Autodesk Fusion 360 part; units mm, degrees
(part 8 of 8)
sketch "Sketch1 (2)" plane through (0, 0, 0) normal (0, 0, 1) x (1, 0, 0) in component "Component"
  spline S0 degree 5 poles (13.0648, -1.7938) (13.065, -1.7938) (13.0653, -1.7938) (13.0658, -1.7939) (13.0667, -1.794) (13.0679, -1.7941) (13.0693, -1.7943) (13.071, -1.7944) (13.0728, -1.7946) (13.0748, -1.7948) (13.077, -1.795) (13.0793, -1.7952) (13.0819, -1.7955) (13.0846, -1.7957) (13.0874, -1.7959) (13.0905, -1.7961) (13.0937, -1.7964) (13.0971, -1.7966) (13.1006, -1.7968) (13.1043, -1.797) (13.1081, -1.7972) (13.1121, -1.7975) (13.1162, -1.7977) (13.1205, -1.7978) (13.1249, -1.798) (13.1295, -1.7982) (13.1342, -1.7984) (13.1391, -1.7985) (13.1441, -1.7987) (13.1492, -1.7988) (13.1544, -1.7989) (13.1598, -1.799) (13.1653, -1.7991) (13.171, -1.7991) (13.1767, -1.7992) (13.1826, -1.7992) (13.1886, -1.7992) (13.1948, -1.7992) (13.201, -1.7991) (13.2074, -1.7991) (13.2139, -1.799) (13.2205, -1.7989) (13.2272, -1.7987) (13.2341, -1.7986) (13.241, -1.7984) (13.2481, -1.7982) (13.2552, -1.798) (13.2625, -1.7977) (13.2699, -1.7974) (13.2774, -1.7971) (13.285, -1.7968) (13.2927, -1.7964) (13.3004, -1.796) (13.3083, -1.7955) (13.3163, -1.7951) (13.3244, -1.7946) (13.3326, -1.7941) (13.3409, -1.7935) (13.3493, -1.7929) (13.3578, -1.7923) (13.3663, -1.7916) (13.375, -1.7909) (13.3838, -1.7902) (13.3926, -1.7895) (13.4015, -1.7887) (13.4106, -1.7878) (13.4197, -1.787) (13.4289, -1.7861) (13.4382, -1.7851) (13.4475, -1.7842) (13.457, -1.7832) (13.4665, -1.7821) (13.4762, -1.781) (13.4859, -1.7799) (13.4957, -1.7787) (13.5055, -1.7775) (13.5155, -1.7763) (13.5255, -1.775) (13.5356, -1.7737) (13.5458, -1.7723) (13.5561, -1.7709) (13.5664, -1.7695) (13.5768, -1.768) (13.5873, -1.7665) (13.5978, -1.7649) (13.6085, -1.7633) (13.6192, -1.7616) (13.63, -1.7599) (13.6408, -1.7582) (13.6517, -1.7564) (13.6627, -1.7546) (13.6738, -1.7527) (13.6849, -1.7508) (13.6961, -1.7489) (13.7074, -1.7469) (13.7187, -1.7448) (13.7301, -1.7428) (13.7415, -1.7406) (13.7531, -1.7384) (13.7647, -1.7362) (13.7763, -1.734) (13.788, -1.7316) (13.7998, -1.7293) (13.8117, -1.7269) (13.8236, -1.7244) (13.8355, -1.7219) (13.8476, -1.7194) (13.8596, -1.7168) (13.8718, -1.7142) (13.884, -1.7115) (13.8963, -1.7088) (13.9086, -1.706) (13.921, -1.7032) (13.9334, -1.7003) (13.9459, -1.6974) (13.9584, -1.6944) (13.971, -1.6914) (13.9837, -1.6883) (13.9964, -1.6852) (14.0092, -1.682) (14.022, -1.6788) (14.0349, -1.6755) (14.0478, -1.6722) (14.0608, -1.6689) (14.0738, -1.6655) (14.0869, -1.662) (14.1, -1.6585) (14.1132, -1.6549) (14.1264, -1.6513) (14.1397, -1.6476) (14.153, -1.6439) (14.1664, -1.6402) (14.1798, -1.6364) (14.1933, -1.6325) (14.2068, -1.6286) (14.2204, -1.6246) (14.234, -1.6206) (14.2476, -1.6165) (14.2613, -1.6124) (14.2751, -1.6082) (14.2889, -1.604) (14.3027, -1.5998) (14.3166, -1.5954) (14.3305, -1.5911) (14.3445, -1.5866) (14.3585, -1.5821) (14.3725, -1.5776) (14.3866, -1.573) (14.4007, -1.5684) (14.4149, -1.5637) (14.4291, -1.559) (14.4434, -1.5542) (14.4577, -1.5493) (14.472, -1.5444) (14.4864, -1.5395) (14.5008, -1.5344) (14.5152, -1.5294) (14.5297, -1.5243) (14.5442, -1.5191) (14.5588, -1.5139) (14.5734, -1.5086) (14.588, -1.5033) (14.6027, -1.4979) (14.6174, -1.4925) (14.6322, -1.487) (14.6469, -1.4814) (14.6617, -1.4758) (14.6766, -1.4702) (14.6915, -1.4645) (14.7064, -1.4587) (14.7213, -1.4529) (14.7363, -1.4471) (14.7513, -1.4411) (14.7664, -1.4352) (14.7814, -1.4291) (14.7965, -1.4231) (14.8117, -1.4169) (14.8269, -1.4107) (14.8421, -1.4045) (14.8573, -1.3982) (14.8725, -1.3918) (14.8878, -1.3854) (14.9032, -1.3789) (14.9185, -1.3724) (14.9339, -1.3659) (14.9493, -1.3592) (14.9647, -1.3525) (14.9802, -1.3458) (14.9957, -1.339) (15.0112, -1.3322) (15.0267, -1.3252) (15.0423, -1.3183) (15.0579, -1.3113) (15.0735, -1.3042) (15.0892, -1.2971) (15.1049, -1.2899) (15.1206, -1.2827) (15.1363, -1.2754) (15.152, -1.268) (15.1678, -1.2606) (15.1836, -1.2532) (15.1994, -1.2456) (15.2153, -1.2381) (15.2311, -1.2304) (15.247, -1.2228) (15.2629, -1.215) (15.2789, -1.2072) (15.2948, -1.1994) (15.3108, -1.1915) (15.3268, -1.1835) (15.3428, -1.1755) (15.3589, -1.1674) (15.3749, -1.1593) (15.391, -1.1511) (15.4071, -1.1429) (15.4232, -1.1346) (15.4394, -1.1262) (15.4555, -1.1178) (15.4717, -1.1094) (15.4879, -1.1008) (15.5041, -1.0923) (15.5204, -1.0836) (15.5366, -1.0749) (15.5529, -1.0662) (15.5692, -1.0574) (15.5855, -1.0485) (15.6018, -1.0396) (15.6182, -1.0307) (15.6345, -1.0216) (15.6509, -1.0126) (15.6673, -1.0034) (15.6837, -0.9942) (15.7001, -0.985) (15.7165, -0.9757) (15.733, -0.9663) (15.7495, -0.9569) (15.7659, -0.9474) (15.7824, -0.9379) (15.7989, -0.9283) (15.8154, -0.9187) (15.832, -0.909) (15.8452, -0.9012) (15.8552, -0.8953) (15.8618, -0.8913) (15.8651, -0.8894) knots 0 0 0 0 0 0 0.00416667 0.00833333 0.0125 0.01666667 0.02083333 0.025 0.02916667 0.03333333 0.0375 0.04166667 0.04583333 0.05 0.05416667 0.05833333 0.0625 0.06666667 0.07083333 0.075 0.07916667 0.08333333 0.0875 0.09166667 0.09583333 0.1 0.10416667 0.10833333 0.1125 0.11666667 0.12083333 0.125 0.12916667 0.13333333 0.1375 0.14166667 0.14583333 0.15 0.15416667 0.15833333 0.1625 0.16666667 0.17083333 0.175 0.17916667 0.18333333 0.1875 0.19166667 0.19583333 0.2 0.20416667 0.20833333 0.2125 0.21666667 0.22083333 0.225 0.22916667 0.23333333 0.2375 0.24166667 0.24583333 0.25 0.25416667 0.25833333 0.2625 0.26666667 0.27083333 0.275 0.27916667 0.28333333 0.2875 0.29166667 0.29583333 0.3 0.30416667 0.30833333 0.3125 0.31666667 0.32083333 0.325 0.32916667 0.33333333 0.3375 0.34166667 0.34583333 0.35 0.35416667 0.35833333 0.3625 0.36666667 0.37083333 0.375 0.37916667 0.38333333 0.3875 0.39166667 0.39583333 0.4 0.40416667 0.40833333 0.4125 0.41666667 0.42083333 0.425 0.42916667 0.43333333 0.4375 0.44166667 0.44583333 0.45 0.45416667 0.45833333 0.4625 0.46666667 0.47083333 0.475 0.47916667 0.48333333 0.4875 0.49166667 0.49583333 0.5 0.50416667 0.50833333 0.5125 0.51666667 0.52083333 0.525 0.52916667 0.53333333 0.5375 0.54166667 0.54583333 0.55 0.55416667 0.55833333 0.5625 0.56666667 0.57083333 0.575 0.57916667 0.58333333 0.5875 0.59166667 0.59583333 0.6 0.60416667 0.60833333 0.6125 0.61666667 0.62083333 0.625 0.62916667 0.63333333 0.6375 0.64166667 0.64583333 0.65 0.65416667 0.65833333 0.6625 0.66666667 0.67083333 0.675 0.67916667 0.68333333 0.6875 0.69166667 0.69583333 0.7 0.70416667 0.70833333 0.7125 0.71666667 0.72083333 0.725 0.72916667 0.73333333 0.7375 0.74166667 0.74583333 0.75 0.75416667 0.75833333 0.7625 0.76666667 0.77083333 0.775 0.77916667 0.78333333 0.7875 0.79166667 0.79583333 0.8 0.80416667 0.80833333 0.8125 0.81666667 0.82083333 0.825 0.82916667 0.83333333 0.8375 0.84166667 0.84583333 0.85 0.85416667 0.85833333 0.8625 0.86666667 0.87083333 0.875 0.87916667 0.88333333 0.8875 0.89166667 0.89583333 0.9 0.90416667 0.90833333 0.9125 0.91666667 0.92083333 0.925 0.92916667 0.93333333 0.9375 0.94166667 0.94583333 0.95 0.95416667 0.95833333 0.9625 0.96666667 0.97083333 0.975 0.97916667 0.98333333 0.9875 0.99166667 0.99583333 1 1 1 1 1 1
  spline S1 degree 5 poles (13.0648, 1.7938) (13.065, 1.7938) (13.0653, 1.7938) (13.0658, 1.7939) (13.0667, 1.794) (13.0679, 1.7941) (13.0693, 1.7943) (13.071, 1.7944) (13.0728, 1.7946) (13.0748, 1.7948) (13.077, 1.795) (13.0793, 1.7952) (13.0819, 1.7955) (13.0846, 1.7957) (13.0874, 1.7959) (13.0905, 1.7961) (13.0937, 1.7964) (13.0971, 1.7966) (13.1006, 1.7968) (13.1043, 1.797) (13.1081, 1.7972) (13.1121, 1.7975) (13.1162, 1.7977) (13.1205, 1.7978) (13.1249, 1.798) (13.1295, 1.7982) (13.1342, 1.7984) (13.1391, 1.7985) (13.1441, 1.7987) (13.1492, 1.7988) (13.1544, 1.7989) (13.1598, 1.799) (13.1653, 1.7991) (13.171, 1.7991) (13.1767, 1.7992) (13.1826, 1.7992) (13.1886, 1.7992) (13.1948, 1.7992) (13.201, 1.7991) (13.2074, 1.7991) (13.2139, 1.799) (13.2205, 1.7989) (13.2272, 1.7987) (13.2341, 1.7986) (13.241, 1.7984) (13.2481, 1.7982) (13.2552, 1.798) (13.2625, 1.7977) (13.2699, 1.7974) (13.2774, 1.7971) (13.285, 1.7968) (13.2927, 1.7964) (13.3004, 1.796) (13.3083, 1.7955) (13.3163, 1.7951) (13.3244, 1.7946) (13.3326, 1.7941) (13.3409, 1.7935) (13.3493, 1.7929) (13.3578, 1.7923) (13.3663, 1.7916) (13.375, 1.7909) (13.3838, 1.7902) (13.3926, 1.7895) (13.4015, 1.7887) (13.4106, 1.7878) (13.4197, 1.787) (13.4289, 1.7861) (13.4382, 1.7851) (13.4475, 1.7842) (13.457, 1.7832) (13.4665, 1.7821) (13.4762, 1.781) (13.4859, 1.7799) (13.4957, 1.7787) (13.5055, 1.7775) (13.5155, 1.7763) (13.5255, 1.775) (13.5356, 1.7737) (13.5458, 1.7723) (13.5561, 1.7709) (13.5664, 1.7695) (13.5768, 1.768) (13.5873, 1.7665) (13.5978, 1.7649) (13.6085, 1.7633) (13.6192, 1.7616) (13.63, 1.7599) (13.6408, 1.7582) (13.6517, 1.7564) (13.6627, 1.7546) (13.6738, 1.7527) (13.6849, 1.7508) (13.6961, 1.7489) (13.7074, 1.7469) (13.7187, 1.7448) (13.7301, 1.7428) (13.7415, 1.7406) (13.7531, 1.7384) (13.7647, 1.7362) (13.7763, 1.734) (13.788, 1.7316) (13.7998, 1.7293) (13.8117, 1.7269) (13.8236, 1.7244) (13.8355, 1.7219) (13.8476, 1.7194) (13.8596, 1.7168) (13.8718, 1.7142) (13.884, 1.7115) (13.8963, 1.7088) (13.9086, 1.706) (13.921, 1.7032) (13.9334, 1.7003) (13.9459, 1.6974) (13.9584, 1.6944) (13.971, 1.6914) (13.9837, 1.6883) (13.9964, 1.6852) (14.0092, 1.682) (14.022, 1.6788) (14.0349, 1.6755) (14.0478, 1.6722) (14.0608, 1.6689) (14.0738, 1.6655) (14.0869, 1.662) (14.1, 1.6585) (14.1132, 1.6549) (14.1264, 1.6513) (14.1397, 1.6476) (14.153, 1.6439) (14.1664, 1.6402) (14.1798, 1.6364) (14.1933, 1.6325) (14.2068, 1.6286) (14.2204, 1.6246) (14.234, 1.6206) (14.2476, 1.6165) (14.2613, 1.6124) (14.2751, 1.6082) (14.2889, 1.604) (14.3027, 1.5998) (14.3166, 1.5954) (14.3305, 1.5911) (14.3445, 1.5866) (14.3585, 1.5821) (14.3725, 1.5776) (14.3866, 1.573) (14.4007, 1.5684) (14.4149, 1.5637) (14.4291, 1.559) (14.4434, 1.5542) (14.4577, 1.5493) (14.472, 1.5444) (14.4864, 1.5395) (14.5008, 1.5344) (14.5152, 1.5294) (14.5297, 1.5243) (14.5442, 1.5191) (14.5588, 1.5139) (14.5734, 1.5086) (14.588, 1.5033) (14.6027, 1.4979) (14.6174, 1.4925) (14.6322, 1.487) (14.6469, 1.4814) (14.6617, 1.4758) (14.6766, 1.4702) (14.6915, 1.4645) (14.7064, 1.4587) (14.7213, 1.4529) (14.7363, 1.4471) (14.7513, 1.4411) (14.7664, 1.4352) (14.7814, 1.4291) (14.7965, 1.4231) (14.8117, 1.4169) (14.8269, 1.4107) (14.8421, 1.4045) (14.8573, 1.3982) (14.8725, 1.3918) (14.8878, 1.3854) (14.9032, 1.3789) (14.9185, 1.3724) (14.9339, 1.3659) (14.9493, 1.3592) (14.9647, 1.3525) (14.9802, 1.3458) (14.9957, 1.339) (15.0112, 1.3322) (15.0267, 1.3252) (15.0423, 1.3183) (15.0579, 1.3113) (15.0735, 1.3042) (15.0892, 1.2971) (15.1049, 1.2899) (15.1206, 1.2827) (15.1363, 1.2754) (15.152, 1.268) (15.1678, 1.2606) (15.1836, 1.2532) (15.1994, 1.2456) (15.2153, 1.2381) (15.2311, 1.2304) (15.247, 1.2228) (15.2629, 1.215) (15.2789, 1.2072) (15.2948, 1.1994) (15.3108, 1.1915) (15.3268, 1.1835) (15.3428, 1.1755) (15.3589, 1.1674) (15.3749, 1.1593) (15.391, 1.1511) (15.4071, 1.1429) (15.4232, 1.1346) (15.4394, 1.1262) (15.4555, 1.1178) (15.4717, 1.1094) (15.4879, 1.1008) (15.5041, 1.0923) (15.5204, 1.0836) (15.5366, 1.0749) (15.5529, 1.0662) (15.5692, 1.0574) (15.5855, 1.0485) (15.6018, 1.0396) (15.6182, 1.0307) (15.6345, 1.0216) (15.6509, 1.0126) (15.6673, 1.0034) (15.6837, 0.9942) (15.7001, 0.985) (15.7165, 0.9757) (15.733, 0.9663) (15.7495, 0.9569) (15.7659, 0.9474) (15.7824, 0.9379) (15.7989, 0.9283) (15.8154, 0.9187) (15.832, 0.909) (15.8452, 0.9012) (15.8552, 0.8953) (15.8618, 0.8913) (15.8651, 0.8894) knots 0 0 0 0 0 0 0.00416667 0.00833333 0.0125 0.01666667 0.02083333 0.025 0.02916667 0.03333333 0.0375 0.04166667 0.04583333 0.05 0.05416667 0.05833333 0.0625 0.06666667 0.07083333 0.075 0.07916667 0.08333333 0.0875 0.09166667 0.09583333 0.1 0.10416667 0.10833333 0.1125 0.11666667 0.12083333 0.125 0.12916667 0.13333333 0.1375 0.14166667 0.14583333 0.15 0.15416667 0.15833333 0.1625 0.16666667 0.17083333 0.175 0.17916667 0.18333333 0.1875 0.19166667 0.19583333 0.2 0.20416667 0.20833333 0.2125 0.21666667 0.22083333 0.225 0.22916667 0.23333333 0.2375 0.24166667 0.24583333 0.25 0.25416667 0.25833333 0.2625 0.26666667 0.27083333 0.275 0.27916667 0.28333333 0.2875 0.29166667 0.29583333 0.3 0.30416667 0.30833333 0.3125 0.31666667 0.32083333 0.325 0.32916667 0.33333333 0.3375 0.34166667 0.34583333 0.35 0.35416667 0.35833333 0.3625 0.36666667 0.37083333 0.375 0.37916667 0.38333333 0.3875 0.39166667 0.39583333 0.4 0.40416667 0.40833333 0.4125 0.41666667 0.42083333 0.425 0.42916667 0.43333333 0.4375 0.44166667 0.44583333 0.45 0.45416667 0.45833333 0.4625 0.46666667 0.47083333 0.475 0.47916667 0.48333333 0.4875 0.49166667 0.49583333 0.5 0.50416667 0.50833333 0.5125 0.51666667 0.52083333 0.525 0.52916667 0.53333333 0.5375 0.54166667 0.54583333 0.55 0.55416667 0.55833333 0.5625 0.56666667 0.57083333 0.575 0.57916667 0.58333333 0.5875 0.59166667 0.59583333 0.6 0.60416667 0.60833333 0.6125 0.61666667 0.62083333 0.625 0.62916667 0.63333333 0.6375 0.64166667 0.64583333 0.65 0.65416667 0.65833333 0.6625 0.66666667 0.67083333 0.675 0.67916667 0.68333333 0.6875 0.69166667 0.69583333 0.7 0.70416667 0.70833333 0.7125 0.71666667 0.72083333 0.725 0.72916667 0.73333333 0.7375 0.74166667 0.74583333 0.75 0.75416667 0.75833333 0.7625 0.76666667 0.77083333 0.775 0.77916667 0.78333333 0.7875 0.79166667 0.79583333 0.8 0.80416667 0.80833333 0.8125 0.81666667 0.82083333 0.825 0.82916667 0.83333333 0.8375 0.84166667 0.84583333 0.85 0.85416667 0.85833333 0.8625 0.86666667 0.87083333 0.875 0.87916667 0.88333333 0.8875 0.89166667 0.89583333 0.9 0.90416667 0.90833333 0.9125 0.91666667 0.92083333 0.925 0.92916667 0.93333333 0.9375 0.94166667 0.94583333 0.95 0.95416667 0.95833333 0.9625 0.96666667 0.97083333 0.975 0.97916667 0.98333333 0.9875 0.99166667 0.99583333 1 1 1 1 1 1
  spline S2 degree 5 poles (13.0636, -1.7936) (13.0637, -1.7936) (13.0638, -1.7936) (13.0639, -1.7936) (13.0641, -1.7937) (13.0644, -1.7937) (13.0646, -1.7937) (13.0647, -1.7937) (13.0648, -1.7938) (13.0648, -1.7938) knots 0 0 0 0 0 0 0.2 0.4 0.6 0.8 1 1 1 1 1 1
  spline S3 degree 5 poles (13.0636, 1.7936) (13.0637, 1.7936) (13.0638, 1.7936) (13.0639, 1.7936) (13.0641, 1.7937) (13.0644, 1.7937) (13.0646, 1.7937) (13.0647, 1.7937) (13.0648, 1.7938) (13.0648, 1.7938) knots 0 0 0 0 0 0 0.2 0.4 0.6 0.8 1 1 1 1 1 1
  line L0 (0, 0) -> (13.0636, -1.7936)
  line L1 (0, 0) -> (13.0636, 1.7936)
  arc A0 (15.8651, -0.8894) -> (15.8651, 0.8894) centre (0, 0) ccw
  point P0 (13.0685, -1.7942)
  point P1 (13.0747, -1.7948)
  point P2 (13.0834, -1.7956)
  point P3 (13.0945, -1.7964)
  point P4 (13.1082, -1.7972)
  point P5 (13.1243, -1.798)
  point P6 (13.1429, -1.7986)
  point P7 (13.164, -1.799)
  point P8 (13.1876, -1.7992)
  point P9 (13.2137, -1.799)
  point P10 (13.2422, -1.7984)
  point P11 (13.2732, -1.7973)
  point P12 (13.3067, -1.7956)
  point P13 (13.3426, -1.7934)
  point P14 (13.381, -1.7904)
  point P15 (13.4218, -1.7868)
  point P16 (13.465, -1.7823)
  point P17 (13.5107, -1.7769)
  point P18 (13.5587, -1.7705)
  point P19 (13.609, -1.7632)
  point P20 (13.6618, -1.7548)
  point P21 (13.7168, -1.7452)
  point P22 (13.7742, -1.7344)
  point P23 (13.8338, -1.7223)
  point P24 (13.8957, -1.7089)
  point P25 (13.9598, -1.6941)
  point P26 (14.0261, -1.6778)
  point P27 (14.0946, -1.6599)
  point P28 (14.1652, -1.6405)
  point P29 (14.2379, -1.6194)
  point P30 (14.3128, -1.5966)
  point P31 (14.3896, -1.572)
  point P32 (14.4685, -1.5456)
  point P33 (14.5494, -1.5173)
  point P34 (14.6321, -1.487)
  point P35 (14.7168, -1.4547)
  point P36 (14.8034, -1.4203)
  point P37 (14.8917, -1.3838)
  point P38 (14.9818, -1.3451)
  point P39 (15.0737, -1.3041)
  point P40 (15.1672, -1.2609)
  point P41 (15.2624, -1.2153)
  point P42 (15.3592, -1.1673)
  point P43 (15.4575, -1.1168)
  point P44 (15.5573, -1.0638)
  point P45 (15.6585, -1.0083)
  point P46 (15.7611, -0.9502)
  point P47 (13.0685, 1.7942)
  point P48 (13.0747, 1.7948)
  point P49 (13.0834, 1.7956)
  point P50 (13.0945, 1.7964)
  point P51 (13.1082, 1.7972)
  point P52 (13.1243, 1.798)
  point P53 (13.1429, 1.7986)
  point P54 (13.164, 1.799)
  point P55 (13.1876, 1.7992)
  point P56 (13.2137, 1.799)
  point P57 (13.2422, 1.7984)
  point P58 (13.2732, 1.7973)
  point P59 (13.3067, 1.7956)
  point P60 (13.3426, 1.7934)
  point P61 (13.381, 1.7904)
  point P62 (13.4218, 1.7868)
  point P63 (13.465, 1.7823)
  point P64 (13.5107, 1.7769)
  point P65 (13.5587, 1.7705)
  point P66 (13.609, 1.7632)
  point P67 (13.6618, 1.7548)
  point P68 (13.7168, 1.7452)
  point P69 (13.7742, 1.7344)
  point P70 (13.8338, 1.7223)
  point P71 (13.8957, 1.7089)
  point P72 (13.9598, 1.6941)
  point P73 (14.0261, 1.6778)
  point P74 (14.0946, 1.6599)
  point P75 (14.1652, 1.6405)
  point P76 (14.2379, 1.6194)
  point P77 (14.3128, 1.5966)
  point P78 (14.3896, 1.572)
  point P79 (14.4685, 1.5456)
  point P80 (14.5494, 1.5173)
  point P81 (14.6321, 1.487)
  point P82 (14.7168, 1.4547)
  point P83 (14.8034, 1.4203)
  point P84 (14.8917, 1.3838)
  point P85 (14.9818, 1.3451)
  point P86 (15.0737, 1.3041)
  point P87 (15.1672, 1.2609)
  point P88 (15.2624, 1.2153)
  point P89 (15.3592, 1.1673)
  point P90 (15.4575, 1.1168)
  point P91 (15.5573, 1.0638)
  point P92 (15.6585, 1.0083)
  point P93 (15.7611, 0.9502)
sketch "Sketch2" plane through (0, 0, 0) normal (0, 0, 1) x (1, 0, 0) in component "Component"
  circle A0 centre (0, 0) radius 10.7825
extrude "Extrude1" add sketch "Sketch2" along normal blind 6 makes body 1 in component "Component"
extrude "Extrude2" add sketch "Sketch1 (2)" along normal blind 6 separate body makes body 2 in component "Component"
pattern_circular "C-Pattern1" count 12 over 360 about axis through (0, 0, 1.75) along (0, 0, 1) of "Extrude2" makes body 3 at (4.0705, 1.6597, 2) makes body 4 at (2.6953, 3.4725, 2) makes body 5 at (0.5979, 4.3549, 2) makes body 6 at (-1.6597, 4.0705, 2) makes body 7 at (-4.0705, 1.6597, 2) makes body 8 at (-4.3549, 0.5979, 2) makes body 9 at (-4.0705, -1.6597, 2) makes body 10 at (-2.6953, -3.4725, 2) makes body 11 at (-0.5979, -4.3549, 2) makes body 12 at (2.6953, -3.4725, 2) makes body 13 at (3.4725, -2.6953, 2) in component "Component"
combine "Combine1" operation add target body 1 tool bodies 2 3 4 5 6 7 8 9 10 11 12 13 in component "Component"
sketch "Sketch3" plane through (0, 0, 0) normal (0, 0, 1) x (1, 0, 0) in component "Component"
  line L0 (0, 0) -> (49.8984, 0) construction
  line L1 (49.8984, 0) -> (49.8984, 3) construction
  line L2 (49.8984, 3) -> (0, 3) construction
  line L3 (0, 3) -> (0, 0) construction
  constraint perpendicular L0 L1
  constraint parallel L0 L2
  constraint parallel L1 L3
extrude "Extrude3" cut sketch "Sketch1" against normal blind 6 contours A24 | A25 | A26 | A27 bodies 1 in component "Component"
component "Component" placed x (1, 0, 0) y (0, 1, 0) z (0, 0, 1) at (0, 0, 0)
component "Component" placed x (1, 0, 0) y (0, 1, 0) z (0, 0, 1) at (34, 0, 0)

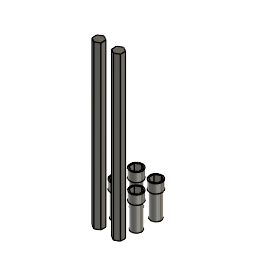
design "card-shuffler-hex-shaft-and-connectors"
part number: 2026-07-29-21-30-18-226
part number: 2026-07-29-22-06-59-016
part number: 2026-07-29-22-06-59-022
part number: 2026-07-29-22-06-59-026
Autodesk Fusion 360 part; units mm, degrees
sketch "Sketch1" plane through (0, 0, 0) normal (0, 0, 1) x (1, 0, 0)
  line L0 (-2.5, -1.4434) -> (0, -2.8868)
  line L1 (0, -2.8868) -> (2.5, -1.4434)
  line L2 (2.5, -1.4434) -> (2.5, 1.4434)
  line L3 (2.5, 1.4434) -> (0, 2.8868)
  line L4 (0, 2.8868) -> (-2.5, 1.4434)
  line L5 (-2.5, 1.4434) -> (-2.5, -1.4434)
  line L6 (-2.65, 8.47) -> (0, 6.94)
  line L7 (0, 6.94) -> (2.65, 8.47)
  line L8 (2.65, 8.47) -> (2.65, 11.53)
  line L9 (2.65, 11.53) -> (0, 13.06)
  line L10 (0, 13.06) -> (-2.65, 11.53)
  line L11 (-2.65, 11.53) -> (-2.65, 8.47)
  circle A0 centre (0, 10) radius 3.5
  point P0 (0, 10)
  dimension "d3" = 2.5
  dimension "d4" = 2.65
  dimension "d5" = 7
  constraint coincident P0 A0.centre
  measures "d3" distance of origin L5
  measures "d4" distance of P0 L11
  measures "d5" diameter of A0
extrude "Extrude1" add sketch "Sketch1" along normal blind 5 contours A0 makes body 1
extrude "Extrude2" add sketch "Sketch1" along normal blind 1 contours L6 L7 L8 L9 L10 L11 bodies 1
sketch "Sketch2" plane through (0, 0, 0) normal (0, 0, 1) x (1, 0, 0)
  circle A0 centre (0, 10) radius 2.9
  dimension "d10" = 5.8
  measures "d10" diameter of A0
extrude "Extrude3" add sketch "Sketch2" against normal blind 14 bodies 1
extrude "Extrude4" add sketch "Sketch1" along normal blind 91 separate body contours L0 L1 L2 L3 L4 L5 makes body 2
move_body "Move1" bodies 1 to x (1, 0, 0) y (0, 1, 0) z (0, 0, 1) at (0, 0, 13)
copy_body "CopyPasteBodies1" bodies 1 makes body 3
move_body "Move2" bodies 3 to x (1, 0, 0) y (0, 1, 0) z (0, 0, 1) at (0, 11, 0)
copy_body "Body->Comp1" bodies 3 removing the originals makes body 4 in component "Component"
copy_body "Body->Comp2" bodies 1 removing the originals makes body 5 in component "Component'"
copy_body "Body->Comp3" bodies 2 removing the originals makes body 6 in component "Component''"
component "Component" placed x (1, 0, 0) y (0, 1, 0) z (0, 0, 1) at (0, 0, 0)
component "Component'" placed x (1, 0, 0) y (0, 1, 0) z (0, 0, 1) at (0, 0, 0)
component "Component''" placed x (1, 0, 0) y (0, 1, 0) z (0, 0, 1) at (0, 0, 0)
component "Component" placed x (1, 0, 0) y (0, 1, 0) z (0, 0, 1) at (-11, 0, 0)
component "Component'" placed x (1, 0, 0) y (0, 1, 0) z (0, 0, 1) at (-11, 0, 0)
component "Component''" placed x (1, 0, 0) y (0, 1, 0) z (0, 0, 1) at (-11, 0, 0)

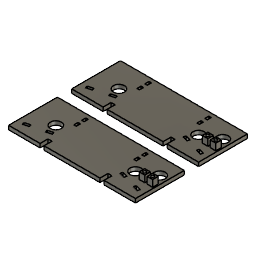
design "card-shuffler-side-plates"
part number: 2026-07-14-13-37-18-342
part number: 2026-07-29-15-30-40-937
Autodesk Fusion 360 part; units mm, degrees
sketch "Sketch1" plane through (0, 0, 0) normal (0, 0, 1) x (1, 0, 0)
  line L0 (0, 0) -> (81, 0)
  line L1 (81, 0) -> (81, 103)
  line L2 (81, 103) -> (0, 103)
  line L3 (0, 103) -> (0, 0)
  line L4 (76, 98) -> (5, 98)
  line L5 (5, 98) -> (5, 5)
  line L6 (5, 5) -> (76, 5)
  line L7 (76, 5) -> (76, 98)
  line L8 (76, 98) -> (5, 5) construction
  line L9 (5, 98) -> (76, 5) construction
  line L10 (81, 0) -> (121, 0)
  line L11 (121, 0) -> (121, 5)
  line L12 (121, 5) -> (81, 5)
  line L13 (81, 5) -> (81, 0)
  line L14 (0, 0) -> (-40, 0)
  line L15 (-40, 0) -> (-40, 5)
  line L16 (-40, 5) -> (0, 5)
  line L17 (0, 5) -> (0, 0)
  line L18 (81, 103) -> (121, 103)
  line L19 (121, 103) -> (121, 98)
  line L20 (121, 98) -> (81, 98)
  line L21 (81, 98) -> (81, 103)
  line L22 (0, 103) -> (-40, 103)
  line L23 (-40, 103) -> (-40, 98)
  line L24 (-40, 98) -> (0, 98)
  line L25 (0, 98) -> (0, 103)
  line L26 (76, 51.5) -> (76, 45)
  line L27 (76, 45) -> (81, 45)
  line L28 (81, 45) -> (81, 58)
  line L29 (81, 58) -> (76, 58)
  line L30 (76, 58) -> (76, 45)
  line L31 (0, 58) -> (5, 58)
  line L32 (5, 58) -> (5, 45)
  line L33 (5, 45) -> (0, 45)
  line L34 (0, 45) -> (0, 58)
  line L35 (81, 98) -> (121, 98)
  line L36 (121, 98) -> (121, 5)
  line L37 (121, 5) -> (81, 5)
  line L38 (81, 5) -> (81, 98)
  line L39 (-40, 98) -> (0, 98)
  line L40 (0, 98) -> (0, 5)
  line L41 (0, 5) -> (-40, 5)
  line L42 (-40, 5) -> (-40, 98)
  line L43 (76, 58) -> (108, 58)
  line L44 (108, 58) -> (108, 45)
  line L45 (108, 45) -> (76, 45)
  line L46 (76, 45) -> (76, 58)
  line L47 (5, 45) -> (-27, 45)
  line L48 (-27, 45) -> (-27, 58)
  line L49 (-27, 58) -> (5, 58)
  line L50 (5, 58) -> (5, 45)
  line L51 (76, 98) -> (81, 98)
  line L52 (5, 98) -> (0, 98)
  line L53 (0, 5) -> (5, 5)
  line L54 (76, 5) -> (81, 5)
  point P0 (40.5, 51.5)
  dimension "d1" = 81
  dimension "d2" = 103
  dimension "d3" = 71
  dimension "d4" = 93
  dimension "d7" = 6.5
  dimension "d8" = 32
  dimension "d9" = 13
  dimension "d14" = 40
  dimension "d15" = 40
  dimension "d16" = 40
  dimension "d17" = 40
  constraint horizontal L0
  constraint vertical L1
  constraint horizontal L2
  constraint vertical L3
  constraint coincident L0.start L3.end
  constraint horizontal L4
  constraint perpendicular L4 L5
  constraint parallel L4 L6
  constraint parallel L5 L7
  constraint coincident L8 P0
  constraint coincident L9 P0
  constraint horizontal L10
  constraint vertical L11
  constraint horizontal L12
  constraint vertical L13
  constraint horizontal L14
  constraint vertical L15
  constraint horizontal L16
  constraint vertical L17
  constraint horizontal L18
  constraint vertical L19
  constraint horizontal L20
  constraint vertical L21
  constraint horizontal L22
  constraint vertical L23
  constraint horizontal L24
  constraint vertical L25
  constraint midpoint L7 L26.start
  constraint parallel L7 L26
  constraint horizontal L27
  constraint vertical L28
  constraint horizontal L29
  constraint vertical L30
  constraint coincident L1 L28.end
  constraint horizontal L31
  constraint vertical L32
  constraint horizontal L33
  constraint vertical L34
  constraint coincident L5 L32.end
  constraint coincident L3 L31.start
  constraint horizontal L35
  constraint vertical L36
  constraint horizontal L37
  constraint vertical L38
  constraint horizontal L39
  constraint vertical L40
  constraint horizontal L41
  constraint vertical L42
  constraint horizontal L43
  constraint vertical L44
  constraint horizontal L45
  constraint vertical L46
  constraint horizontal L47
  constraint vertical L48
  constraint horizontal L49
  constraint vertical L50
  measures "d1" distance of L0.start L0.end
  measures "d2" distance of L0.start L2.end
  measures "d3" distance of L5.end L6.end
  measures "d4" distance of L4.end L5.end
  measures "d7" distance of L26.start L26.end
  measures "d8" distance of L32.end L47.end
  measures "d9" distance of L32.end L31.end
  measures "d14" distance of L36 L38
  measures "d15" distance of L3 L42
  measures "d16" distance of L15 L17
  measures "d17" distance of L19 L21
extrude "Extrude1" add sketch "Sketch1" along normal blind 62 contours L0 L1 L3 L6 L13 L17 L53 L54 | L3 L14 L15 L16 L17 L41 | L1 L10 L11 L12 L13 L37 makes body 1
sketch "Sketch2" plane through (0, 0, 62) normal (0, 0, 1) x (-1, 0, 0)
  line L0 (-76, -98) -> (-81, -98)
  line L1 (-5, -98) -> (0, -98)
  line L2 (0, -5) -> (-5, -5)
  line L3 (40, -98) -> (-121, -98)
  line L4 (-121, -98) -> (-121, -103)
  line L5 (-121, -103) -> (40, -103)
  line L6 (40, -103) -> (40, -98)
  line L7 (40, -5) -> (-121, -5)
  line L8 (-121, -5) -> (-121, 0)
  line L9 (-121, 0) -> (40, 0)
  line L10 (40, 0) -> (40, -5)
  line L11 (0, -5) -> (40, -5)
  line L12 (40, -5) -> (40, 0)
  line L13 (40, 0) -> (-121, 0)
  line L14 (-121, 0) -> (-121, -5)
  line L15 (-121, -5) -> (-81, -5)
  line L16 (-81, -5) -> (-76, -5)
  line L17 (-76, -5) -> (-5, -5)
  line L18 (-5, -5) -> (0, -5)
  constraint horizontal L3
  constraint vertical L4
  constraint horizontal L5
  constraint vertical L6
  constraint horizontal L7
  constraint vertical L8
  constraint horizontal L9
  constraint vertical L10
sketch "Sketch5" plane through (0, 0, 0) normal (0, -1, 0) x (1, 0, 0)
  line L0 (-9.2177, 45.8096) -> (-9.9941, 42.9118)
  line L1 (-9.9941, 42.9118) -> (-3.2327, 41.1001)
  line L2 (-2.4562, 43.9979) -> (-3.2327, 41.1001)
  line L3 (-9.2177, 45.8096) -> (-2.4562, 43.9979)
  line L4 (-32.3999, 52.0213) -> (-33.1764, 49.1235)
  line L5 (-26.4149, 47.3118) -> (-33.1764, 49.1235)
  line L6 (-32.3999, 52.0213) -> (-25.6384, 50.2095)
  line L7 (-25.6384, 50.2095) -> (-26.4149, 47.3118)
  line L8 (-40, 0) -> (121, 0)
  line L9 (121, 0) -> (121, 62)
  line L10 (121, 62) -> (-40, 62)
  line L11 (-40, 62) -> (-40, 0)
  line L12 (90.2177, 45.8096) -> (83.4562, 43.9979)
  line L13 (90.2177, 45.8096) -> (90.9942, 42.9118)
  line L14 (90.9942, 42.9118) -> (84.2327, 41.1001)
  line L15 (83.4562, 43.9979) -> (84.2327, 41.1001)
  line L16 (106.6384, 50.2095) -> (107.4149, 47.3118)
  line L17 (107.4149, 47.3118) -> (114.1764, 49.1235)
  line L18 (113.3999, 52.0213) -> (114.1764, 49.1235)
  line L19 (113.3999, 52.0213) -> (106.6384, 50.2095)
  line L20 (4, 10) -> (1, 10)
  line L21 (1, 10) -> (1, 5)
  line L22 (1, 5) -> (4, 5)
  line L23 (4, 5) -> (4, 10)
  line L24 (1, 15) -> (4, 15)
  line L25 (4, 15) -> (4, 20)
  line L26 (4, 20) -> (1, 20)
  line L27 (1, 20) -> (1, 15)
  line L28 (77, 15) -> (77, 20)
  line L29 (77, 20) -> (80, 20)
  line L30 (80, 20) -> (80, 15)
  line L31 (80, 15) -> (77, 15)
  line L32 (77, 10) -> (80, 10)
  line L33 (80, 10) -> (80, 5)
  line L34 (80, 5) -> (77, 5)
  line L35 (77, 5) -> (77, 10)
  circle A0 centre (111, 21.25) radius 7
  circle A1 centre (116, 35.25) radius 1.9
  circle A2 centre (106, 35.25) radius 1.9
  line L36 (119.5, 38.75) -> (112.5, 38.75)
  line L37 (112.5, 38.75) -> (112.5, 31.75)
  line L38 (112.5, 31.75) -> (119.5, 31.75)
  line L39 (119.5, 31.75) -> (119.5, 38.75)
  line L40 (119.5, 38.75) -> (112.5, 31.75) construction
  line L41 (112.5, 38.75) -> (119.5, 31.75) construction
  line L42 (109.5, 38.75) -> (102.5, 38.75)
  line L43 (102.5, 38.75) -> (102.5, 31.75)
  line L44 (102.5, 31.75) -> (109.5, 31.75)
  line L45 (109.5, 31.75) -> (109.5, 38.75)
  line L46 (109.5, 38.75) -> (102.5, 31.75) construction
  line L47 (102.5, 38.75) -> (109.5, 31.75) construction
  point P0 (116, 35.25)
  point P1 (106, 35.25)
  dimension "d54" = 14
  dimension "d55" = 10
  dimension "d56" = 21.25
  dimension "d59" = 3.8
  dimension "d60" = 14
  dimension "d61" = 5
  dimension "d62" = 3.8
  dimension "d63" = 10
  dimension "d64" = 7
  dimension "d65" = 7
  dimension "d66" = 7
  dimension "d67" = 7
  constraint perpendicular L5 L7
  constraint horizontal L20
  constraint vertical L21
  constraint horizontal L22
  constraint vertical L23
  constraint horizontal L24
  constraint vertical L25
  constraint horizontal L26
  constraint vertical L27
  constraint horizontal L36
  constraint perpendicular L36 L37
  constraint parallel L36 L38
  constraint parallel L37 L39
  constraint coincident L40 P0
  constraint coincident L41 P0
  constraint coincident P0 A1.centre
  constraint horizontal L42
  constraint perpendicular L42 L43
  constraint parallel L42 L44
  constraint parallel L43 L45
  constraint coincident L46 P1
  constraint coincident L47 P1
  constraint coincident P1 A2.centre
  measures "d54" diameter of A0
  measures "d55" distance of L9 A0.centre
  measures "d56" distance of L8 A0.centre
  measures "d59" diameter of A1
  measures "d60" vertical distance of A0.centre P0
  measures "d61" distance of L9 P0
  measures "d62" diameter of A2
  measures "d63" distance of P0 P1
  measures "d64" distance of L37.end L38.end
  measures "d65" distance of L36.end L37.end
  measures "d66" distance of L43.end L44.end
  measures "d67" distance of L42.end L43.end
sketch "Sketch3" plane through (0, 0, 0) normal (0, -1, 0) x (1, 0, 0)
  line L0 (-40, 0) -> (121, 0)
  circle A0 centre (91, 32) radius 7
  line L1 (40.5, 82) -> (40.5, 0)
  circle A1 centre (-10, 32) radius 7
  line L2 (81, 0) -> (121, 0)
  line L3 (0, 0) -> (-40, 0)
  line L4 (121, 0) -> (121, 62)
  line L5 (121, 62) -> (-40, 62)
  line L6 (-40, 62) -> (-40, 0)
  dimension "d22" = 14
  dimension "d23" = 50.5
  dimension "d24" = 14
  dimension "d25" = 50.5
  dimension "d26" = 32
  dimension "d27" = 32
  constraint midpoint L0 L1.end
  measures "d22" diameter of A0
  measures "d23" distance of A0.centre L1
  measures "d24" diameter of A1
  measures "d25" distance of L1 A1.centre
  measures "d26" distance of A0.centre L2
  measures "d27" distance of A1.centre L3
ref_plane "WorkPlane2" through (40.5, 2.5, 31) normal (1, 0, 0) x (0, 1, 0)
extrude "Extrude10" cut sketch "Sketch3" against normal blind 5 contours A0 | A1 bodies 1
extrude "Extrude12" cut sketch "Sketch5" against normal blind 28 contours L0 L1 L2 L3 | L4 L5 L6 L7 | L12 L13 L14 L15 | L16 L17 L18 L19 | L20 L21 L22 L23 | L24 L25 L26 L27 | L28 L29 L30 L31 | L32 L33 L34 L35 | A0 | A1 | A2 bodies 1
delete_face "DeleteFace1" 1 faces at (78, 5, 48) on bodies 1
delete_face "DeleteFace2" 1 faces at (2, 5, 48) on bodies 1
copy_body "Body->Comp2" bodies 1 removing the originals makes body 2 in component "Component"
extrude "Extrude2" add sketch "Sketch5" against normal blind 13.5 contours L36 L37 L38 L39 | L42 L43 L44 L45 bodies 2 in component "Component"
sketch "Sketch8" plane through (0, 0, 62) normal (0, 0, 1) x (-1, 0, 0)
  line L0 (-121, -5) -> (40, -5)
  line L1 (40, -5) -> (40, 0)
  line L2 (40, 0) -> (-121, 0)
  line L3 (-121, 0) -> (-121, -5)
  line L4 (-81, 0) -> (-76, 0)
  line L5 (-76, 0) -> (-76, -5)
  line L6 (-76, -5) -> (-81, -5)
  line L7 (-81, -5) -> (-81, 0)
  line L8 (0, 0) -> (-5, 0)
  line L9 (-5, 0) -> (-5, -5)
  line L10 (-5, -5) -> (0, -5)
  line L11 (0, -5) -> (0, 0)
  constraint horizontal L4
  constraint vertical L5
  constraint horizontal L6
  constraint vertical L7
  constraint coincident L0 L5.end
  constraint coincident L2 L4.start
  constraint horizontal L8
  constraint vertical L9
  constraint horizontal L10
  constraint vertical L11
  constraint coincident L0 L9.end
  constraint coincident L8.start L11.end
extrude "Extrude3" cut sketch "Sketch8" against normal blind 10 contours L0 L2 L4 L5 L6 L7 | L0 L2 L8 L9 L10 L11 bodies 2 in component "Component"
component "Component" placed x (1, 0, 0) y (0, 0, 1) z (0, -1, 0) at (0, 34.0061, 0.0547)
component "Component" placed x (1, 0, 0) y (0, 0, 1) z (0, -1, 0) at (0, 114.0061, 0.0547)
equation "d5 = 42.00 mm + 20 mm"
equation "d56 = 23.25 mm + 3 mm - 5 mm"
equation "d74 = -5 mm - 8.5 mm"

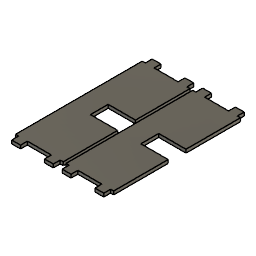
design "card-shuffler-platforms"
part number: 2026-07-28-16-04-37-564
part number: 2026-07-29-15-19-14-329
part number: 2026-07-29-15-19-15-565
Autodesk Fusion 360 part; units mm, degrees
sketch "Sketch1" plane through (0, 0, 0) normal (0, 0, 1) x (1, 0, 0)
  line L0 (0, 0) -> (35, 0)
  line L1 (35, 0) -> (35, 103)
  line L2 (35, 103) -> (0, 103)
  line L3 (0, 103) -> (0, 0)
  line L4 (0, 0) -> (2.25, 0)
  line L5 (2.25, 0) -> (8.75, 0)
  line L6 (8.75, 0) -> (8.75, 5)
  line L7 (8.75, 5) -> (2.25, 5)
  line L8 (2.25, 5) -> (2.25, 0)
  line L9 (32.75, 0) -> (26.25, 0)
  line L10 (26.25, 0) -> (26.25, 5)
  line L11 (26.25, 5) -> (32.75, 5)
  line L12 (32.75, 5) -> (32.75, 0)
  line L13 (32.75, 103) -> (26.25, 103)
  line L14 (26.25, 103) -> (26.25, 98)
  line L15 (26.25, 98) -> (32.75, 98)
  line L16 (32.75, 98) -> (32.75, 103)
  line L17 (2.25, 103) -> (8.75, 103)
  line L18 (8.75, 103) -> (8.75, 98)
  line L19 (8.75, 98) -> (2.25, 98)
  line L20 (2.25, 98) -> (2.25, 103)
  line L21 (0, 5) -> (35, 5)
  line L22 (0, 98) -> (35, 98)
  line L23 (17.5, 0) -> (17.5, 5)
  line L24 (17.5, 98) -> (17.5, 103)
  line L25 (55, 58) -> (15, 58)
  line L26 (15, 58) -> (15, 45)
  line L27 (15, 45) -> (55, 45)
  line L28 (55, 45) -> (55, 58)
  line L29 (55, 58) -> (15, 45) construction
  line L30 (15, 58) -> (55, 45) construction
  point P0 (35, 51.5)
  dimension "d1" = 35
  dimension "d2" = 103
  dimension "d5" = 2.25
  dimension "d7" = 2.25
  dimension "d8" = 8.75
  dimension "d9" = 8.75
  dimension "d10" = 2.25
  dimension "d11" = 2.25
  dimension "d12" = 8.75
  dimension "d13" = 8.75
  dimension "d14" = 40
  dimension "d15" = 13
  constraint horizontal L0
  constraint vertical L1
  constraint horizontal L2
  constraint vertical L3
  constraint coincident L0.start L3.end
  constraint coincident L0 L4.end
  constraint horizontal L5
  constraint vertical L6
  constraint horizontal L7
  constraint vertical L8
  constraint horizontal L9
  constraint vertical L10
  constraint horizontal L11
  constraint vertical L12
  constraint coincident L0 L9.start
  constraint horizontal L13
  constraint vertical L14
  constraint horizontal L15
  constraint vertical L16
  constraint coincident L2 L13.start
  constraint horizontal L17
  constraint vertical L18
  constraint horizontal L19
  constraint vertical L20
  constraint coincident L2 L17.start
  constraint coincident L3 L21.start
  constraint coincident L1 L21.end
  constraint perpendicular L1 L21
  constraint coincident L3 L22.start
  constraint coincident L1 L22.end
  constraint perpendicular L1 L22
  constraint midpoint L0 L23.start
  constraint midpoint L21 L23.end
  constraint midpoint L22 L24.start
  constraint midpoint L2 L24.end
  constraint horizontal L25
  constraint perpendicular L25 L26
  constraint parallel L25 L27
  constraint parallel L26 L28
  constraint coincident L29 P0
  constraint coincident L30 P0
  constraint midpoint L1 P0
  measures "d1" distance of L0.start L0.end
  measures "d2" distance of L0.start L2.end
  measures "d5" distance of L3 L8
  measures "d7" distance of L1 L12
  measures "d8" distance of L6 L23
  measures "d9" distance of L10 L23
  measures "d10" distance of L1 L16
  measures "d11" distance of L3 L20
  measures "d12" distance of L14 L24
  measures "d13" distance of L18 L24
  measures "d14" distance of L26.end L27.end
  measures "d15" distance of L25.end L26.end
extrude "Extrude1" add sketch "Sketch1" along normal blind 2.5 contours L0 L5 L6 L7 L8 L21 | L1 L3 L7 L11 L15 L19 L21 L22 L25 L26 L27 | L2 L17 L18 L19 L20 L22 | L0 L9 L10 L11 L12 L21 | L2 L13 L14 L15 L16 L22 makes body 1
copy_body "CopyPasteBodies1" bodies 1 makes body 2
move_body "Move1" bodies 2 to x (1, 0, 0) y (0, 1, 0) z (0, 0, 1) at (37, 0, 0)
copy_body "Body->Comp1" bodies 1 removing the originals makes body 3 in component "Component"
copy_body "Body->Comp2" bodies 2 removing the originals makes body 4 in component "Component'"
component "Component" placed x (1, 0, 0) y (0, 1, 0) z (0, 0, 1) at (0, 0, 0)
component "Component'" placed x (1, 0, 0) y (0, 1, 0) z (0, 0, 1) at (0, 0, 0)
equation "d1 = 17 mm + 7 mm + 7 mm + 4 mm"
equation "d7 = 2.00 mm + 0.25 mm"
equation "d8 = 8.5 mm + 0.25 mm"
equation "d9 = 8.5 mm + 0.25 mm"
